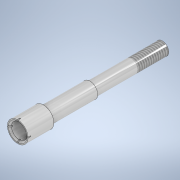
# Autodesk Inventor part: PINO DO BLOCO DE CONTATO
Saved by Autodesk Inventor 2022 (Build 260153000, 153)
## iProperties
Created: 2023-07-19
Part Number: PINO DO BLOCO DE CONTATO
Material: Aluminum 6061-AHC
Document SubType Name: Modeling
Designer: Usuário
Density: 2.7 g/cm^3
Appearance: Aluminum - Dark
Author: Usuário
Autodesk Inventor part; units mm, degrees
ref_plane "YZ Plane" through (0, 0, 0) normal (1, 0, 0) x (0, 1, 0)
ref_plane "XZ Plane" through (0, 0, 0) normal (0, 1, 0) x (-1, 0, 0)
ref_plane "XY Plane" through (0, 0, 0) normal (0, 0, 1) x (1, 0, 0)
sketch "Sketch1" plane through (0, 0, 0) normal (1, 0, 0) x (0, 1, 0)
  line L0 (0, 0) -> (0, -28) construction
  line L1 (0, 0) -> (2, 0)
  line L2 (2, 0) -> (2, -5)
  line L3 (2, -5) -> (0, -5)
  line L4 (0, -5) -> (0, 0)
  line L5 (0, -5) -> (1.5, -5)
  line L6 (1.5, -5) -> (1.5, -14)
  line L7 (1.5, -14) -> (0, -14)
  line L8 (0, -14) -> (0, -5)
  line L9 (0, -14) -> (1.25, -14)
  line L10 (1.25, -14) -> (1.25, -28)
  line L11 (1.25, -28) -> (0, -28)
  line L12 (0, -28) -> (0, -14)
  line L13 (1.5, -4) -> (1.5, 0)
  line L14 (0, -4) -> (1.5, -4)
  line L15 (2, 0) -> (1.5, 0)
  line L16 (0, -4) -> (0, -5)
  dimension "d0" = 28
  dimension "d2" = 5
  dimension "d5" = 9
  dimension "d6" = 3
  dimension "d7" = 1.25
  dimension "d23" = 4
  dimension "d24" = 0.5
  constraints: 34 end point, 6 parallel, 3 horizontal, 3 perpendicular, 2 collinear, 2 point on line, 1 vertical
  measures "d0" distance of L0.start L0.end
  measures "d2" distance of L1.end L2.end
  measures "d5" distance of L5.end L6.end
  measures "d6" diameter of L6 L0
  measures "d7" distance of L10.end L11.end
  measures "d23" diameter of L2 L0
  measures "d24" distance between parallel lines of L13 L2
revolve "Revolution1" add sketch "Sketch1" angle 360 about axis through (0, 0, 0) along (0, 0, -1) contours L1 L2 L3 L4 L14 L13 | L3 L6 L7 L8 | L7 L10 L11 L12
sketch "Sketch2" plane through (0, 0, 0) normal (0, 0, 1) x (1, 0, 0)
  line L0 (0, 0) -> (0, 5.9662) construction
  circle A0 centre (0, 0) radius 2 projected
  line L1 (0, 0) -> (0, -6.6565) construction
  line L2 (0, 0) -> (4.6514, 0) construction
  line L3 (0, 0) -> (-5.9334, 0) construction
  line L4 (1.9984, -0.08) -> (1.4967, -0.1)
  line L5 (0.1, -1.9975) -> (0.1, -1.4967)
  line L6 (1.4967, -0.1) -> (1.9984, -0.08)
  circle A1 centre (0, 0) radius 1.5 projected
  line L7 (0.1, 1.4967) -> (0.1, 1.9975)
  line L8 (-0.1, 1.4967) -> (-0.1, 1.9975)
  line L9 (-1.4967, 0.1) -> (-1.9984, 0.08)
  line L10 (-1.4967, -0.1) -> (-1.9984, -0.08)
  line L11 (-0.08, -1.9984) -> (-0.1, -1.4967)
  line L12 (1.4967, 0.1) -> (1.9984, 0.08)
  line L13 (1.9984, 0.08) -> (1.4967, 0.1)
  dimension "d14" = 0.1
  constraints: 28 end point, 2 horizontal, 2 parallel, 2 vertical, 18 other
  measures "d14" distance between parallel lines of L1 L5
extrude "Extrusion1" cut sketch "Sketch2" against normal blind 0.5 contours A0 L4 A1 L12 | L7 A1 L8 A0 | A0 L11 A1 L5 | L9 A1 L10 A0
chamfer "Chamfer1" distance 0.3 angle 45 4 edges at (1.0607, 1.0607, 0) (-1.0607, 1.0607, 0) (-1.0607, -1.0607, 0) (1.0607, -1.0607, 0)
thread "Thread1" size "M2.5x0.45" class "6g" standard "ANSI Metric M Profile" length 6 offset 8
body "Solid1"
